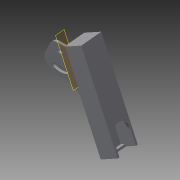
# Autodesk Inventor part: camera-holder
Saved by Autodesk Inventor 2014 (Build 180170000, 170)
## iProperties
Created: 2017-09-09
Part Number: camera-holder
Material: 一般
Document SubType Name: Modeling
Designer: hide
Density: 1 g/cm^3
Appearance: 既定
Author: hide
Autodesk Inventor part; units mm, degrees
ref_plane "YZ Plane" through (0, 0, 0) normal (1, 0, 0) x (0, 1, 0)
ref_plane "XZ Plane" through (0, 0, 0) normal (0, 1, 0) x (-1, 0, 0)
ref_plane "XY Plane" through (0, 0, 0) normal (0, 0, 1) x (1, 0, 0)
sketch "スケッチ1" plane through (0, 0, 0) normal (0, 1, 0) x (-1, 0, 0)
  circle A0 centre (0, 0) radius 1.5
  arc A1 (-3.5392, -9.3528) -> (3.3007, -9.4396) centre (0, 0) ccw construction
  arc A2 (-4.0701, -10.7557) -> (3.7958, -10.8555) centre (0, 0) ccw
  arc A3 (-3.0083, -7.9498) -> (2.8056, -8.0236) centre (0, 0) ccw
  arc A4 (-3.0083, -7.9498) -> (-4.0701, -10.7557) centre (-3.5392, -9.3528) ccw
  arc A5 (3.7958, -10.8555) -> (2.8056, -8.0236) centre (3.3007, -9.4396) ccw
  line L0 (-3, 3.6775) -> (5, 3.6775)
  line L1 (5, 3.6775) -> (11, -8.9445)
  line L2 (11, -8.9445) -> (5, -14)
  line L3 (5, -14) -> (-5, -14)
  line L4 (-5, -14) -> (-9, -9.4181)
  line L5 (-9, -9.4181) -> (-3, 3.6775)
  line L6 (-9, -9.4181) -> (-12.4157, -16.8734)
  line L7 (-12.4157, -16.8734) -> (-5, -14)
  dimension "d0" = 3
  dimension "d1" = 40
  dimension "d2" = 1.5
  dimension "d3" = 8.5
  dimension "d4" = 8
  dimension "d5" = 3
  dimension "d6" = 10
  dimension "d7" = 5
  dimension "d8" = 14
  dimension "d9" = 20
  dimension "d10" = 9
  constraints: 16 end point, 10 point on circle, 6 centre point, 4 tangent, 2 coincident, 1 collinear, 1 horizontal, 1 parallel
  measures "d0" diameter of A0
  measures "d2" radius of A4
  measures "d3" radius of A3
  measures "d4" distance of L0.start L0.end
  measures "d5" horizontal distance of point (0, 0) L0.start
  measures "d6" distance of L2.end L3.end
  measures "d7" horizontal distance of point (0, 0) L3.end
  measures "d8" distance from line of point (0, 0) L3
  measures "d9" horizontal distance of L1.end L4.end
  measures "d10" horizontal distance of point (0, 0) L4.end
extrude "押し出し1" add sketch "スケッチ1" along normal blind 1.5
ref_plane "作業平面2" through (9, 1.5, -9.4181) normal (0.8953108, 0.1736482, 0.410201) x (0.4165291, 0, -0.9091224)
sketch "スケッチ5" plane through (9, 1.5, -9.4181) normal (0.8953108, 0.1736482, 0.410201) x (0.4165291, 0, -0.9091224)
  line L0 (-14.4048, -1.4772) -> (8.2005, -1.4772) projected
  line L1 (-14.4048, 0) -> (8.2005, 0) projected
  line L2 (-14.4048, -1.4772) -> (-14.4048, 0) projected
  line L3 (-14.4048, -1.4772) -> (40.5952, -1.4772)
  line L4 (40.5952, -1.4772) -> (40.5952, 13.7228)
  line L5 (40.5952, 13.7228) -> (-14.4048, 13.7228)
  line L6 (-14.4048, 13.7228) -> (-14.4048, -1.4772)
  line L7 (8.2005, -1.4772) -> (8.2005, 0) projected
  point P0 (-12.311, -0.7376)
  dimension "d24" = 15.2
  dimension "d25" = 55
  constraints: 8 end point, 2 parallel, 1 horizontal, 1 perpendicular
  measures "d24" distance of L5.end L0.start
  measures "d25" distance of L0.start L3.end
extrude "押し出し4" add sketch "スケッチ5" along normal blind 1 and the other way blind 0.5
fillet "フィレット1" radius 5 3 edges at (-11, 0.75, -8.9445) (-5, 0.75, -14) (-5, 0.75, 3.6775)
sketch "スケッチ6" plane through (9.8953, 1.6736, -9.0079) normal (0.8953108, 0.1736482, 0.410201) x (0.4165291, 0, -0.9091224)
  line L0 (37.489, 7.9172) -> (33.989, 7.9172)
  line L1 (33.989, 7.9172) -> (33.989, 4.4172)
  line L2 (33.989, 4.4172) -> (37.489, 4.4172)
  line L3 (37.489, 4.4172) -> (37.489, 7.9172)
  point P0 (-12.311, -0.7376)
  dimension "d31" = 3.5
  dimension "d32" = 3.5
  constraints: 8 end point, 2 parallel, 1 horizontal, 1 perpendicular
  measures "d31" distance of L0.start L0.end
  measures "d32" distance of L0.end L1.end
extrude "押し出し5" cut sketch "スケッチ6" against normal blind 2
sketch "スケッチ7" plane through (9.8953, 1.6736, -9.0079) normal (0.8953108, 0.1736482, 0.410201) x (0.4165291, 0, -0.9091224)
  line L0 (-14.4048, -1.4772) -> (40.5952, -1.4772) projected
  line L1 (40.5952, -1.4772) -> (40.5952, 13.7228) projected
  line L2 (-14.4048, 13.7228) -> (40.5952, 13.7228)
  line L3 (40.5952, 13.7228) -> (40.5952, 12.4228)
  line L4 (40.5952, 12.4228) -> (-14.4048, 12.4228)
  line L5 (-14.4048, 12.4228) -> (-14.4048, 13.7228)
  line L6 (-14.4048, -1.4772) -> (40.5952, -1.4772)
  line L7 (40.5952, -1.4772) -> (40.5952, -0.1772)
  line L8 (40.5952, -0.1772) -> (-14.4048, -0.1772)
  line L9 (-14.4048, -0.1772) -> (-14.4048, -1.4772)
  line L10 (40.5952, -1.4772) -> (39.2952, -1.4772)
  line L11 (39.2952, -1.4772) -> (39.2952, 13.7228)
  line L12 (39.2952, 13.7228) -> (40.5952, 13.7228)
  line L13 (40.5952, 13.7228) -> (40.5952, -1.4772)
  line L14 (-14.4048, 13.7228) -> (-13.1048, 13.7228)
  line L15 (-13.1048, 13.7228) -> (-13.1048, -1.4772)
  line L16 (-13.1048, -1.4772) -> (-14.4048, -1.4772)
  line L17 (-14.4048, -1.4772) -> (-14.4048, 13.7228)
  point P0 (-12.311, -0.7376)
  dimension "d35" = 1.3
  dimension "d36" = 1.3
  dimension "d37" = 1.3
  dimension "d38" = 1.3
  constraints: 32 end point, 8 parallel, 4 horizontal, 4 perpendicular, 4 point on line
  measures "d35" distance between parallel lines of L2 L4
  measures "d36" distance between parallel lines of L8 L0
  measures "d37" distance between parallel lines of L13 L11
  measures "d38" distance between parallel lines of L17 L15
extrude "押し出し6" add sketch "スケッチ7" along normal blind 7 contours L9 L8 L15 L0 | L15 L8 L11 L0 | L17 L4 L15 L8 | L11 L8 L1 L0 | L5 L2 L15 L4 | L15 L2 L11 L4 | L11 L2 L1 L4
sketch "スケッチ8" plane through (16.1625, 2.8892, -6.1365) normal (0.8953108, 0.1736482, 0.410201) x (0.4165291, 0, -0.9091224)
  line L0 (-14.4048, -1.4772) -> (40.5952, -1.4772) projected
  line L1 (40.5952, -1.4772) -> (40.5952, -0.1772) projected
  line L2 (40.5952, -0.1772) -> (-13.1048, -0.1772) projected
  line L3 (-13.1048, -0.1772) -> (-13.1048, 12.4228) projected
  line L4 (-13.1048, 12.4228) -> (40.5952, 12.4228) projected
  line L5 (40.5952, 12.4228) -> (40.5952, 13.7228) projected
  line L6 (40.5952, 13.7228) -> (-14.4048, 13.7228) projected
  line L7 (-14.4048, 13.7228) -> (-14.4048, -1.4772) projected
  line L8 (-14.4048, 13.7228) -> (26.4511, 13.7228)
  line L9 (26.4511, 13.7228) -> (26.4511, -1.4772)
  line L10 (26.4511, -1.4772) -> (-14.4048, -1.4772)
  line L11 (-14.4048, -1.4772) -> (-14.4048, 13.7228)
  point P0 (-12.311, -0.7376)
  constraints: 8 end point, 2 parallel, 1 horizontal, 1 perpendicular, 1 point on line
extrude "押し出し7" add sketch "スケッチ8" along normal blind 1.5
fillet "フィレット2" radius 5.8 2 edges at (25.8904, 15.2535, -30.7747) (27.8796, 2.8449, -29.8633)
sketch "スケッチ9" plane through (25.6946, -0.0416, -46.4224) normal (0.4165291, 0, -0.9091224) x (-0.8953108, -0.1736482, -0.410201)
  line L0 (0, 15.2) -> (-10, 15.2) projected
  line L1 (0, 0) -> (-4.0966, 0)
  line L2 (-4.0966, 0) -> (-4.0966, 15.2)
  line L3 (-4.0966, 15.2) -> (0, 15.2)
  line L4 (0, 15.2) -> (0, 0)
  point P0 (3.9549, 0.7396)
  constraints: 8 end point, 2 parallel, 1 horizontal, 1 perpendicular, 1 point on line
extrude "押し出し8" add sketch "スケッチ9" against normal blind 1.2
fillet "フィレット3" radius 5.8 2 edges at (5, 0.75, -14) (11.9136, 0.75, -16.6788)
equation "\"d7\" = 0.5 * d6"
equation "\"d32\" = d31"
equation "\"d36\" = d35"
equation "\"d37\" = d35"
equation "\"d38\" = d35"
